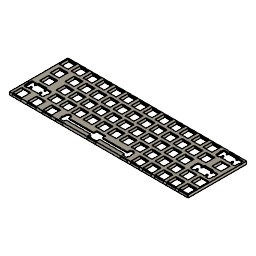
Plate (Autodesk Fusion 360 design; units mm, degrees)
Autodesk Fusion 360 part; units mm, degrees
(part 1 of 2)
sketch "b27d7a26cd9df215f168af8e672502c9323f781d_switch" plane through (0, 0, 0) normal (0, 0, 1) x (1, 0, 0)
  line L0 (271.224, 49.9939) -> (271.224, 54.6929)
  line L1 (255.699, 49.9939) -> (255.699, 53.2225)
  line L2 (248.95, 53.2225) -> (248.95, 49.9939)
  line L3 (255.699, 40.9236) -> (255.699, 45.394)
  line L4 (248.95, 47.1921) -> (248.95, 40.9236)
  line L5 (283.13, 21.6435) -> (269.131, 21.6435)
  line L6 (257.223, 40.6922) -> (271.224, 40.6922)
  line L7 (248.126, 47.1921) -> (248.95, 47.1921)
  line L8 (23.5755, 40.6922) -> (9.576, 40.6922)
  line L9 (35.7699, 40.6922) -> (35.7699, 54.6929)
  line L10 (272.749, 49.9939) -> (271.224, 49.9939)
  line L11 (68.8178, 40.6922) -> (54.8171, 40.6922)
  line L12 (206.93, 21.6435) -> (192.931, 21.6435)
  line L13 (279.499, 49.9939) -> (279.499, 53.2225)
  line L14 (280.325, 47.1921) -> (280.325, 49.9939)
  line L15 (277.774, 40.9236) -> (279.499, 40.9236)
  line L16 (277.774, 39.7221) -> (277.774, 40.9236)
  line L17 (9.576, 54.6929) -> (23.5755, 54.6929)
  line L18 (250.675, 39.7221) -> (253.974, 39.7221)
  line L19 (106.918, 54.6929) -> (106.918, 40.6922)
  line L20 (271.224, 45.394) -> (272.749, 45.394)
  line L21 (87.8678, 40.6922) -> (73.8685, 40.6922)
  line L22 (274.475, 40.9236) -> (274.475, 39.7221)
  line L23 (106.918, 40.6922) -> (92.9185, 40.6922)
  line L24 (271.224, 54.6929) -> (257.223, 54.6929)
  line L25 (253.974, 40.9236) -> (255.699, 40.9236)
  line L26 (253.974, 39.7221) -> (253.974, 40.9236)
  line L27 (274.475, 39.7221) -> (277.774, 39.7221)
  line L28 (257.223, 49.9939) -> (255.699, 49.9939)
  line L29 (272.749, 40.9236) -> (274.475, 40.9236)
  line L30 (248.95, 40.9236) -> (250.675, 40.9236)
  line L31 (68.8178, 54.6929) -> (68.8178, 40.6922)
  line L32 (250.081, 21.6435) -> (250.081, 35.6429)
  line L33 (279.499, 53.2225) -> (272.749, 53.2225)
  line L34 (279.499, 40.9236) -> (279.499, 47.1921)
  line L35 (87.8678, 54.6929) -> (87.8678, 40.6922)
  line L36 (271.224, 40.6922) -> (271.224, 45.394)
  line L37 (73.8685, 40.6922) -> (73.8685, 54.6929)
  line L38 (23.5755, 54.6929) -> (23.5755, 40.6922)
  line L39 (272.749, 45.394) -> (272.749, 40.9236)
  line L40 (264.08, 35.6429) -> (264.08, 21.6435)
  line L41 (280.325, 49.9939) -> (279.499, 49.9939)
  line L42 (225.982, 21.6435) -> (211.981, 21.6435)
  line L43 (54.8171, 54.6929) -> (68.8178, 54.6929)
  line L44 (92.9185, 54.6929) -> (106.918, 54.6929)
  line L45 (73.8685, 54.6929) -> (87.8678, 54.6929)
  line L46 (257.223, 54.6929) -> (257.223, 49.9939)
  line L47 (272.749, 53.2225) -> (272.749, 49.9939)
  line L48 (255.699, 53.2225) -> (248.95, 53.2225)
  line L49 (264.08, 21.6435) -> (250.081, 21.6435)
  line L50 (279.499, 47.1921) -> (280.325, 47.1921)
  line L51 (283.13, 35.6429) -> (283.13, 21.6435)
  line L52 (255.699, 45.394) -> (257.223, 45.394)
  line L53 (49.7692, 40.6922) -> (35.7699, 40.6922)
  line L54 (9.576, 40.6922) -> (9.576, 54.6929)
  line L55 (35.7699, 54.6929) -> (49.7692, 54.6929)
  line L56 (49.7692, 54.6929) -> (49.7692, 40.6922)
  line L57 (248.126, 49.9939) -> (248.126, 47.1921)
  line L58 (269.131, 35.6429) -> (283.13, 35.6429)
  line L59 (54.8171, 40.6922) -> (54.8171, 54.6929)
  line L60 (257.223, 45.394) -> (257.223, 40.6922)
  line L61 (250.675, 40.9236) -> (250.675, 39.7221)
  line L62 (269.131, 21.6435) -> (269.131, 35.6429)
  line L63 (248.95, 49.9939) -> (248.126, 49.9939)
  line L64 (216.455, 73.7429) -> (216.455, 59.7436)
  line L65 (258.862, 65.0709) -> (259.559, 64.7153)
  line L66 (278.368, 59.7436) -> (264.368, 59.7436)
  line L67 (23.4583, 65.6237) -> (24.0123, 65.0709)
  line L68 (126.256, 59.7436) -> (126.256, 73.7429)
  line L69 (258.309, 65.6237) -> (258.862, 65.0709)
  line L70 (216.455, 59.7436) -> (202.456, 59.7436)
  line L71 (25.4827, 64.5915) -> (26.2544, 64.7153)
  line L72 (164.356, 73.7429) -> (178.357, 73.7429)
  line L73 (178.357, 59.7436) -> (164.356, 59.7436)
  line L74 (183.406, 73.7429) -> (197.407, 73.7429)
  line L75 (183.406, 59.7436) -> (183.406, 73.7429)
  line L76 (24.7082, 64.7153) -> (25.4827, 64.5915)
  line L77 (27.9811, 67.0913) -> (27.8598, 67.8656)
  line L78 (257.954, 66.3208) -> (258.309, 65.6237)
  line L79 (264.368, 73.7429) -> (278.368, 73.7429)
  line L80 (240.556, 59.7436) -> (240.556, 73.7429)
  line L81 (240.556, 73.7429) -> (254.555, 73.7429)
  line L82 (202.456, 73.7429) -> (216.455, 73.7429)
  line L83 (26.9517, 65.0709) -> (27.5029, 65.6237)
  line L84 (221.506, 59.7436) -> (221.506, 73.7429)
  line L85 (25.4827, 69.5925) -> (24.7082, 69.4711)
  line L86 (257.831, 67.0913) -> (257.954, 66.3208)
  line L87 (258.309, 68.5631) -> (257.954, 67.8656)
  line L88 (121.205, 73.7429) -> (121.205, 59.7436)
  line L89 (221.506, 73.7429) -> (235.507, 73.7429)
  line L90 (23.1042, 67.8656) -> (22.9829, 67.0913)
  line L91 (259.559, 69.4711) -> (258.862, 69.1155)
  line L92 (235.507, 73.7429) -> (235.507, 59.7436)
  line L93 (23.4583, 68.5631) -> (23.1042, 67.8656)
  line L94 (257.954, 67.8656) -> (257.831, 67.0913)
  line L95 (235.507, 59.7436) -> (221.506, 59.7436)
  line L96 (164.356, 59.7436) -> (164.356, 73.7429)
  line L97 (159.305, 73.7429) -> (159.305, 59.7436)
  line L98 (254.555, 73.7429) -> (254.555, 59.7436)
  line L99 (24.0123, 65.0709) -> (24.7082, 64.7153)
  line L100 (26.2544, 69.4711) -> (25.4827, 69.5925)
  line L101 (26.2544, 64.7153) -> (26.9517, 65.0709)
  line L102 (27.5029, 68.5631) -> (26.9517, 69.1155)
  line L103 (258.862, 69.1155) -> (258.309, 68.5631)
  line L104 (24.0123, 69.1155) -> (23.4583, 68.5631)
  line L105 (197.407, 73.7429) -> (197.407, 59.7436)
  line L106 (24.7082, 69.4711) -> (24.0123, 69.1155)
  line L107 (178.357, 73.7429) -> (178.357, 59.7436)
  line L108 (259.559, 64.7153) -> (260.332, 64.5915)
  line L109 (23.1042, 66.3208) -> (23.4583, 65.6237)
  line L110 (251.331, 91.3239) -> (251.331, 88.0939)
  line L111 (121.205, 59.7436) -> (107.206, 59.7436)
  line L112 (254.555, 59.7436) -> (240.556, 59.7436)
  line L113 (27.8598, 67.8656) -> (27.5029, 68.5631)
  line L114 (273.605, 92.7929) -> (259.606, 92.7929)
  line L115 (197.407, 59.7436) -> (183.406, 59.7436)
  line L116 (140.257, 73.7429) -> (140.257, 59.7436)
  line L117 (261.104, 69.4711) -> (260.332, 69.5925)
  line L118 (26.9517, 69.1155) -> (26.2544, 69.4711)
  line L119 (251.331, 85.2936) -> (251.331, 79.0222)
  line L120 (276.856, 79.0222) -> (276.856, 77.8235)
  line L121 (281.88, 88.0939) -> (281.88, 91.3239)
  line L122 (35.4817, 78.7936) -> (21.4809, 78.7936)
  line L123 (258.08, 79.0222) -> (258.08, 83.494)
  line L124 (54.5317, 92.7929) -> (54.5317, 78.7936)
  line L125 (202.456, 59.7436) -> (202.456, 73.7429)
  line L126 (280.155, 79.0222) -> (281.88, 79.0222)
  line L127 (126.256, 73.7429) -> (140.257, 73.7429)
  line L128 (275.131, 88.0939) -> (273.605, 88.0939)
  line L129 (264.368, 59.7436) -> (264.368, 73.7429)
  line L130 (251.331, 79.0222) -> (253.056, 79.0222)
  line L131 (22.9829, 67.0913) -> (23.1042, 66.3208)
  line L132 (2.4309, 78.7936) -> (2.4309, 92.7929)
  line L133 (273.605, 78.7936) -> (273.605, 83.494)
  line L134 (256.355, 79.0222) -> (258.08, 79.0222)
  line L135 (107.206, 59.7436) -> (107.206, 73.7429)
  line L136 (259.606, 83.494) -> (259.606, 78.7936)
  line L137 (280.155, 77.8235) -> (280.155, 79.0222)
  line L138 (140.257, 59.7436) -> (126.256, 59.7436)
  line L139 (40.531, 92.7929) -> (54.5317, 92.7929)
  line L140 (281.88, 85.2936) -> (282.706, 85.2936)
  line L141 (278.368, 73.7429) -> (278.368, 59.7436)
  line L142 (35.4817, 92.7929) -> (35.4817, 78.7936)
  line L143 (275.131, 79.0222) -> (276.856, 79.0222)
  line L144 (256.355, 77.8235) -> (256.355, 79.0222)
  line L145 (259.606, 92.7929) -> (259.606, 88.0939)
  line L146 (21.4809, 78.7936) -> (21.4809, 92.7929)
  line L147 (145.306, 73.7429) -> (159.305, 73.7429)
  line L148 (145.306, 59.7436) -> (145.306, 73.7429)
  line L149 (27.5029, 65.6237) -> (27.8598, 66.3208)
  line L150 (27.8598, 66.3208) -> (27.9811, 67.0913)
  line L151 (282.706, 85.2936) -> (282.706, 88.0939)
  line L152 (262.354, 65.6237) -> (262.708, 66.3208)
  line L153 (54.5317, 78.7936) -> (40.531, 78.7936)
  line L154 (159.305, 59.7436) -> (145.306, 59.7436)
  line L155 (282.706, 88.0939) -> (281.88, 88.0939)
  line L156 (16.4317, 92.7929) -> (16.4317, 78.7936)
  line L157 (250.507, 88.0939) -> (250.507, 85.2936)
  line L158 (281.88, 79.0222) -> (281.88, 85.2936)
  line L159 (258.08, 91.3239) -> (251.331, 91.3239)
  line L160 (16.4317, 78.7936) -> (2.4309, 78.7936)
  line L161 (258.08, 83.494) -> (259.606, 83.494)
  line L162 (281.88, 91.3239) -> (275.131, 91.3239)
  line L163 (261.801, 65.0709) -> (262.354, 65.6237)
  line L164 (276.856, 77.8235) -> (280.155, 77.8235)
  line L165 (2.4309, 92.7929) -> (16.4317, 92.7929)
  line L166 (250.507, 85.2936) -> (251.331, 85.2936)
  line L167 (262.354, 68.5631) -> (261.801, 69.1155)
  line L168 (273.605, 83.494) -> (275.131, 83.494)
  line L169 (259.606, 88.0939) -> (258.08, 88.0939)
  line L170 (261.104, 64.7153) -> (261.801, 65.0709)
  line L171 (173.881, 92.7929) -> (187.882, 92.7929)
  line L172 (135.781, 78.7936) -> (135.781, 92.7929)
  line L173 (225.982, 78.7936) -> (211.981, 78.7936)
  line L174 (130.732, 92.7929) -> (130.732, 78.7936)
  line L175 (187.882, 78.7936) -> (173.881, 78.7936)
  line L176 (273.605, 88.0939) -> (273.605, 92.7929)
  line L177 (259.606, 78.7936) -> (273.605, 78.7936)
  line L178 (245.032, 92.7929) -> (245.032, 78.7936)
  line L179 (168.83, 92.7929) -> (168.83, 78.7936)
  line L180 (261.801, 69.1155) -> (261.104, 69.4711)
  line L181 (59.581, 78.7936) -> (59.581, 92.7929)
  line L182 (260.332, 69.5925) -> (259.559, 69.4711)
  line L183 (149.782, 78.7936) -> (135.781, 78.7936)
  line L184 (73.5803, 92.7929) -> (73.5803, 78.7936)
  line L185 (262.708, 66.3208) -> (262.832, 67.0913)
  line L186 (262.708, 67.8656) -> (262.354, 68.5631)
  line L187 (40.531, 78.7936) -> (40.531, 92.7929)
  line L188 (78.631, 78.7936) -> (78.631, 92.7929)
  line L189 (111.682, 78.7936) -> (97.681, 78.7936)
  line L190 (78.631, 92.7929) -> (92.6317, 92.7929)
  line L191 (97.681, 78.7936) -> (97.681, 92.7929)
  line L192 (21.4809, 92.7929) -> (35.4817, 92.7929)
  line L193 (59.581, 92.7929) -> (73.5803, 92.7929)
  line L194 (258.08, 88.0939) -> (258.08, 91.3239)
  line L195 (253.056, 79.0222) -> (253.056, 77.8235)
  line L196 (206.93, 78.7936) -> (192.931, 78.7936)
  line L197 (130.732, 78.7936) -> (116.731, 78.7936)
  line L198 (275.131, 91.3239) -> (275.131, 88.0939)
  line L199 (275.131, 83.494) -> (275.131, 79.0222)
  line L200 (73.5803, 78.7936) -> (59.581, 78.7936)
  line L201 (251.331, 88.0939) -> (250.507, 88.0939)
  line L202 (260.332, 64.5915) -> (261.104, 64.7153)
  line L203 (231.031, 92.7929) -> (245.032, 92.7929)
  line L204 (154.831, 92.7929) -> (168.83, 92.7929)
  line L205 (154.831, 78.7936) -> (154.831, 92.7929)
  line L206 (187.882, 92.7929) -> (187.882, 78.7936)
  line L207 (253.056, 77.8235) -> (256.355, 77.8235)
  line L208 (192.931, 92.7929) -> (206.93, 92.7929)
  line L209 (211.981, 92.7929) -> (225.982, 92.7929)
  line L210 (192.931, 78.7936) -> (192.931, 92.7929)
  line L211 (111.682, 92.7929) -> (111.682, 78.7936)
  line L212 (262.832, 67.0913) -> (262.708, 67.8656)
  line L213 (149.782, 92.7929) -> (149.782, 78.7936)
  line L214 (116.731, 92.7929) -> (130.732, 92.7929)
  line L215 (211.981, 78.7936) -> (211.981, 92.7929)
  line L216 (97.681, 92.7929) -> (111.682, 92.7929)
  line L217 (173.881, 78.7936) -> (173.881, 92.7929)
  line L218 (206.93, 92.7929) -> (206.93, 78.7936)
  line L219 (116.731, 78.7936) -> (116.731, 92.7929)
  line L220 (231.031, 78.7936) -> (231.031, 92.7929)
  line L221 (225.982, 92.7929) -> (225.982, 78.7936)
  line L222 (92.6317, 92.7929) -> (92.6317, 78.7936)
  line L223 (92.6317, 78.7936) -> (78.631, 78.7936)
  line L224 (168.83, 78.7936) -> (154.831, 78.7936)
  line L225 (135.781, 92.7929) -> (149.782, 92.7929)
  line L226 (245.032, 78.7936) -> (231.031, 78.7936)
  line L227 (50.056, 73.7429) -> (64.0567, 73.7429)
  line L228 (130.859, 46.9209) -> (130.983, 47.6913)
  line L229 (126.46, 49.1613) -> (126.103, 48.4657)
  line L230 (64.0567, 73.7429) -> (64.0567, 59.7436)
  line L231 (169.12, 54.6929) -> (183.119, 54.6929)
  line L232 (127.71, 45.314) -> (128.483, 45.1915)
  line L233 (183.119, 40.6922) -> (169.12, 40.6922)
  line L234 (125.969, 40.6922) -> (111.967, 40.6922)
  line L235 (102.157, 59.7436) -> (88.156, 59.7436)
  line L236 (145.018, 54.6929) -> (145.018, 40.6922)
  line L237 (221.219, 40.6922) -> (207.22, 40.6922)
  line L238 (21.1942, 59.7436) -> (7.1947, 59.7436)
  line L239 (128.483, 45.1915) -> (129.255, 45.314)
  line L240 (102.157, 73.7429) -> (102.157, 59.7436)
  line L241 (130.859, 48.4657) -> (130.504, 49.1613)
  line L242 (127.012, 45.671) -> (127.71, 45.314)
  line L243 (202.168, 40.6922) -> (188.168, 40.6922)
  line L244 (127.71, 50.0712) -> (127.012, 49.7156)
  line L245 (107.206, 73.7429) -> (121.205, 73.7429)
  line L246 (130.983, 47.6913) -> (130.859, 48.4657)
  line L247 (150.068, 54.6929) -> (164.068, 54.6929)
  line L248 (164.068, 40.6922) -> (150.068, 40.6922)
  line L249 (240.269, 54.6929) -> (240.269, 40.6922)
  line L250 (69.106, 59.7436) -> (69.106, 73.7429)
  line L251 (83.1067, 73.7429) -> (83.1067, 59.7436)
  line L252 (111.967, 54.6929) -> (125.969, 54.6929)
  line L253 (88.156, 59.7436) -> (88.156, 73.7429)
  line L254 (83.1067, 59.7436) -> (69.106, 59.7436)
  line L255 (88.156, 73.7429) -> (102.157, 73.7429)
  line L256 (226.27, 40.6922) -> (226.27, 54.6929)
  line L257 (131.018, 54.6929) -> (145.018, 54.6929)
  line L258 (92.9185, 40.6922) -> (92.9185, 54.6929)
  line L259 (126.103, 48.4657) -> (125.983, 47.6913)
  line L260 (31.0059, 73.7429) -> (45.0053, 73.7429)
  line L261 (50.056, 59.7436) -> (50.056, 73.7429)
  line L262 (69.106, 73.7429) -> (83.1067, 73.7429)
  line L263 (164.068, 54.6929) -> (164.068, 40.6922)
  line L264 (125.983, 47.6913) -> (126.103, 46.9209)
  line L265 (150.068, 40.6922) -> (150.068, 54.6929)
  line L266 (145.018, 40.6922) -> (131.018, 40.6922)
  line L267 (183.119, 54.6929) -> (183.119, 40.6922)
  line L268 (126.103, 46.9209) -> (126.46, 46.222)
  line L269 (130.504, 49.1613) -> (129.952, 49.7156)
  line L270 (64.0567, 59.7436) -> (50.056, 59.7436)
  line L271 (221.219, 54.6929) -> (221.219, 40.6922)
  line L272 (129.255, 50.0712) -> (128.483, 50.1908)
  line L273 (125.969, 54.6929) -> (125.969, 40.6922)
  line L274 (131.018, 40.6922) -> (131.018, 54.6929)
  line L275 (129.255, 45.314) -> (129.952, 45.671)
  line L276 (129.952, 49.7156) -> (129.255, 50.0712)
  line L277 (45.0053, 73.7429) -> (45.0053, 59.7436)
  line L278 (226.27, 54.6929) -> (240.269, 54.6929)
  line L279 (21.1942, 73.7429) -> (21.1942, 59.7436)
  line L280 (111.967, 40.6922) -> (111.967, 54.6929)
  line L281 (188.168, 40.6922) -> (188.168, 54.6929)
  line L282 (207.22, 40.6922) -> (207.22, 54.6929)
  line L283 (240.269, 40.6922) -> (226.27, 40.6922)
  line L284 (188.168, 54.6929) -> (202.168, 54.6929)
  line L285 (130.504, 46.222) -> (130.859, 46.9209)
  line L286 (127.012, 49.7156) -> (126.46, 49.1613)
  line L287 (7.1947, 59.7436) -> (7.1947, 73.7429)
  line L288 (45.0053, 59.7436) -> (31.0059, 59.7436)
  line L289 (7.1947, 73.7429) -> (21.1942, 73.7429)
  line L290 (128.483, 50.1908) -> (127.71, 50.0712)
  line L291 (5.6169, 37.0237) -> (5.971, 37.7197)
  line L292 (184.284, 16.3477) -> (182.5589, 16.3477)
  line L293 (3.5953, 40.9924) -> (0.0951, 40.9924)
  line L294 (0.0951, 95.3477) -> (285.469, 95.3477)
  line L295 (279.592, 37.7197) -> (279.947, 37.0237)
  line L296 (207.22, 54.6929) -> (221.219, 54.6929)
  line L297 (279.947, 37.0237) -> (280.5, 36.4698)
  line L298 (281.969, 40.9924) -> (281.196, 40.87)
  line L299 (279.592, 39.2659) -> (279.469, 38.4941)
  line L300 (137.909, 2.5783) -> (137.909, 7.2775)
  line L301 (281.969, 35.9929) -> (285.469, 35.9929)
  line L302 (6.095, 38.4926) -> (5.971, 39.2659)
  line L303 (285.469, 35.9929) -> (285.469, 0.2288)
  line L304 (285.469, 0.2288) -> (0.0951, 0.2288)
  line L305 (285.469, 95.3477) -> (285.469, 40.9924)
  line L306 (177.5346, 4.0473) -> (184.284, 4.0473)
  line L307 (5.6169, 39.963) -> (5.0629, 40.5158)
  line L308 (279.469, 38.4941) -> (279.592, 37.7197)
  line L309 (5.0629, 36.4698) -> (5.6169, 37.0237)
  line L310 (184.284, 4.0473) -> (184.284, 7.2775)
  line L311 (279.947, 39.963) -> (279.592, 39.2659)
  line L312 (281.196, 40.87) -> (280.5, 40.5158)
  line L313 (31.0059, 59.7436) -> (31.0059, 73.7429)
  line L314 (202.168, 54.6929) -> (202.168, 40.6922)
  line L315 (184.284, 7.2775) -> (185.1095, 7.2775)
  line L316 (280.5, 36.4698) -> (281.196, 36.1142)
  line L317 (3.5939, 35.9929) -> (4.367, 36.1142)
  line L318 (169.12, 40.6922) -> (169.12, 54.6929)
  line L319 (184.284, 10.0776) -> (184.284, 16.3477)
  line L320 (0.0951, 0.2288) -> (0.0951, 35.9929)
  line L321 (280.5, 40.5158) -> (279.947, 39.963)
  line L322 (281.196, 36.1142) -> (281.969, 35.9929)
  line L323 (0.0951, 40.9924) -> (0.0951, 95.3477)
  line L324 (4.367, 36.1142) -> (5.0629, 36.4698)
  line L325 (285.469, 40.9924) -> (281.969, 40.9924)
  line L326 (5.971, 39.2659) -> (5.6169, 39.963)
  line L327 (182.5589, 16.3477) -> (182.5589, 17.548)
  line L328 (5.971, 37.7197) -> (6.095, 38.4926)
  line L329 (129.952, 45.671) -> (130.504, 46.222)
  line L330 (126.46, 46.222) -> (127.012, 45.671)
  line L331 (137.909, 16.5778) -> (123.91, 16.5778)
  line L332 (123.91, 16.5778) -> (123.91, 11.8773)
  line L333 (84.284, 11.8773) -> (84.284, 16.3477)
  line L334 (137.909, 7.2775) -> (177.5346, 7.2775)
  line L335 (82.56, 17.548) -> (79.26, 17.548)
  line L336 (79.26, 17.548) -> (79.26, 16.3477)
  line L337 (4.367, 40.87) -> (3.5953, 40.9924)
  line L338 (77.534, 10.0776) -> (76.71, 10.0776)
  line L339 (76.71, 10.0776) -> (76.71, 7.2775)
  line L340 (84.284, 4.0473) -> (84.284, 7.2775)
  line L341 (4.8121, 16.593) -> (18.813, 16.593)
  line L342 (18.813, 16.593) -> (18.813, 2.5935)
  line L343 (4.8121, 2.5935) -> (4.8121, 16.593)
  line L344 (123.91, 2.5783) -> (137.909, 2.5783)
  line L345 (192.931, 2.5935) -> (206.93, 2.5935)
  line L346 (84.284, 16.3477) -> (82.56, 16.3477)
  line L347 (245.032, 16.593) -> (245.032, 2.5935)
  line L348 (211.981, 16.593) -> (225.982, 16.593)
  line L349 (76.71, 7.2775) -> (77.534, 7.2775)
  line L350 (77.534, 7.2775) -> (77.534, 4.0473)
  line L351 (123.91, 11.8773) -> (84.284, 11.8773)
  line L352 (177.5346, 7.2775) -> (177.5346, 4.0473)
  line L353 (77.534, 4.0473) -> (84.284, 4.0473)
  line L354 (84.284, 7.2775) -> (123.91, 7.2775)
  line L355 (18.813, 2.5935) -> (4.8121, 2.5935)
  line L356 (0.0951, 35.9929) -> (3.5939, 35.9929)
  line L357 (123.91, 7.2775) -> (123.91, 2.5783)
  line L358 (192.931, 11.0133) -> (192.804, 11.2627)
  line L359 (245.032, 2.5935) -> (231.031, 2.5935)
  line L360 (5.0629, 40.5158) -> (4.367, 40.87)
  line L361 (179.2597, 16.3477) -> (177.5346, 16.3477)
  line L362 (82.56, 16.3477) -> (82.56, 17.548)
  line L363 (137.909, 11.8773) -> (137.909, 16.5778)
  line L364 (79.26, 16.3477) -> (77.534, 16.3477)
  line L365 (177.5346, 16.3477) -> (177.5346, 11.8773)
  line L366 (77.534, 16.3477) -> (77.534, 10.0776)
  line L367 (182.5589, 17.548) -> (179.2597, 17.548)
  line L368 (179.2597, 17.548) -> (179.2597, 16.3477)
  line L369 (177.5346, 11.8773) -> (137.909, 11.8773)
  line L370 (231.031, 2.5935) -> (231.031, 16.593)
  line L371 (250.081, 2.5935) -> (250.081, 16.593)
  line L372 (269.131, 16.593) -> (283.13, 16.593)
  line L373 (269.131, 2.5935) -> (269.131, 16.593)
  line L374 (10.4317, 34.174) -> (3.6821, 34.174)
  line L375 (2.8567, 28.1437) -> (3.6821, 28.1437)
  line L376 (11.9558, 30.9425) -> (10.4317, 30.9425)
  line L377 (66.4379, 16.593) -> (66.4379, 2.5935)
  line L378 (3.6821, 28.1437) -> (3.6821, 21.8736)
  line L379 (3.6821, 21.8736) -> (5.406, 21.8736)
  line L380 (10.4317, 26.344) -> (11.9558, 26.344)
  line L381 (10.4317, 21.8736) -> (10.4317, 26.344)
  line L382 (264.08, 16.593) -> (264.08, 2.5935)
  line L383 (189.312, 7.7694) -> (190.008, 7.4152)
  line L384 (2.8567, 30.9425) -> (2.8567, 28.1437)
  line L385 (42.624, 16.593) -> (42.624, 2.5935)
  line L386 (250.081, 16.593) -> (264.08, 16.593)
  line L387 (283.13, 16.593) -> (283.13, 2.5935)
  line L388 (189.312, 11.8139) -> (188.758, 11.2627)
  line L389 (206.93, 2.5935) -> (206.93, 16.593)
  line L390 (188.758, 8.3234) -> (189.312, 7.7694)
  line L391 (5.406, 20.6733) -> (8.7065, 20.6733)
  line L392 (8.7065, 20.6733) -> (8.7065, 21.8736)
  line L393 (225.982, 2.5935) -> (211.981, 2.5935)
  line L394 (28.6246, 16.593) -> (42.624, 16.593)
  line L395 (28.6246, 2.5935) -> (28.6246, 16.593)
  line L396 (10.4317, 30.9425) -> (10.4317, 34.174)
  line L397 (11.9558, 26.344) -> (11.9558, 21.6435)
  line L398 (190.781, 12.2921) -> (190.008, 12.1708)
  line L399 (190.008, 12.1708) -> (189.312, 11.8139)
  line L400 (188.758, 11.2627) -> (188.404, 10.564)
  line L401 (192.252, 11.8139) -> (191.554, 12.1708)
  line L402 (32.5052, 20.6733) -> (32.5052, 21.8736)
  line L403 (25.9553, 30.9425) -> (25.9553, 35.6429)
  line L404 (42.624, 2.5935) -> (28.6246, 2.5935)
  line L405 (192.804, 11.2627) -> (192.252, 11.8139)
  line L406 (245.032, 21.6435) -> (231.031, 21.6435)
  line L407 (52.4372, 16.593) -> (66.4379, 16.593)
  line L408 (192.252, 7.7694) -> (192.804, 8.3234)
  line L409 (192.931, 8.5728) -> (192.931, 2.5935)
  line L410 (188.281, 9.7923) -> (188.404, 9.0193)
  line L411 (188.404, 9.0193) -> (188.758, 8.3234)
  line L412 (264.08, 2.5935) -> (250.081, 2.5935)
  line L413 (211.981, 2.5935) -> (211.981, 16.593)
  line L414 (190.008, 7.4152) -> (190.781, 7.2926)
  line L415 (8.7065, 21.8736) -> (10.4317, 21.8736)
  line L416 (191.554, 12.1708) -> (190.781, 12.2921)
  line L417 (225.982, 16.593) -> (225.982, 2.5935)
  line L418 (66.4379, 2.5935) -> (52.4372, 2.5935)
  line L419 (3.6821, 34.174) -> (3.6821, 30.9425)
  line L420 (231.031, 16.593) -> (245.032, 16.593)
  line L421 (5.406, 21.8736) -> (5.406, 20.6733)
  line L422 (283.13, 2.5935) -> (269.131, 2.5935)
  line L423 (3.6821, 30.9425) -> (2.8567, 30.9425)
  line L424 (190.781, 7.2926) -> (191.554, 7.4152)
  line L425 (192.931, 16.593) -> (192.931, 11.0133)
  line L426 (191.554, 7.4152) -> (192.252, 7.7694)
  line L427 (211.981, 21.6435) -> (211.981, 35.6429)
  line L428 (192.804, 8.3234) -> (192.931, 8.5728)
  line L429 (245.032, 35.6429) -> (245.032, 21.6435)
  line L430 (188.404, 10.564) -> (188.281, 9.7923)
  line L431 (52.4372, 2.5935) -> (52.4372, 16.593)
  line L432 (206.93, 16.593) -> (192.931, 16.593)
  line L433 (11.9558, 35.6429) -> (11.9558, 30.9425)
  line L434 (173.881, 21.6435) -> (173.881, 35.6429)
  line L435 (34.2319, 28.1437) -> (35.0559, 28.1437)
  line L436 (225.982, 35.6429) -> (225.982, 21.6435)
  line L437 (154.831, 35.6429) -> (168.83, 35.6429)
  line L438 (116.731, 21.6435) -> (116.731, 35.6429)
  line L439 (135.781, 35.6429) -> (149.782, 35.6429)
  line L440 (35.0559, 30.9425) -> (34.2319, 30.9425)
  line L441 (40.531, 21.6435) -> (40.531, 35.6429)
  line L442 (135.781, 21.6435) -> (135.781, 35.6429)
  line L443 (54.5317, 35.6429) -> (54.5317, 21.6435)
  line L444 (34.2319, 21.8736) -> (34.2319, 28.1437)
  line L445 (173.881, 35.6429) -> (187.882, 35.6429)
  line L446 (27.4808, 34.174) -> (27.4808, 30.9425)
  line L447 (73.5803, 35.6429) -> (73.5803, 21.6435)
  line L448 (231.031, 35.6429) -> (245.032, 35.6429)
  line L449 (27.4808, 26.344) -> (27.4808, 21.8736)
  line L450 (97.681, 35.6429) -> (111.682, 35.6429)
  line L451 (187.882, 21.6435) -> (173.881, 21.6435)
  line L452 (250.081, 35.6429) -> (264.08, 35.6429)
  line L453 (130.732, 21.6435) -> (116.731, 21.6435)
  line L454 (59.581, 35.6429) -> (73.5803, 35.6429)
  line L455 (73.5803, 21.6435) -> (59.581, 21.6435)
  line L456 (78.631, 35.6429) -> (92.6317, 35.6429)
  line L457 (92.6317, 21.6435) -> (78.631, 21.6435)
  line L458 (168.83, 35.6429) -> (168.83, 21.6435)
  line L459 (29.2062, 21.8736) -> (29.2062, 20.6733)
  line L460 (29.2062, 20.6733) -> (32.5052, 20.6733)
  line L461 (27.4808, 21.8736) -> (29.2062, 21.8736)
  line L462 (92.6317, 35.6429) -> (92.6317, 21.6435)
  line L463 (111.682, 35.6429) -> (111.682, 21.6435)
  line L464 (231.031, 21.6435) -> (231.031, 35.6429)
  line L465 (35.0559, 28.1437) -> (35.0559, 30.9425)
  line L466 (11.9558, 21.6435) -> (25.9553, 21.6435)
  line L467 (154.831, 21.6435) -> (154.831, 35.6429)
  line L468 (78.631, 21.6435) -> (78.631, 35.6429)
  line L469 (97.681, 21.6435) -> (97.681, 35.6429)
  line L470 (149.782, 35.6429) -> (149.782, 21.6435)
  line L471 (168.83, 21.6435) -> (154.831, 21.6435)
  line L472 (25.9553, 35.6429) -> (11.9558, 35.6429)
  line L473 (32.5052, 21.8736) -> (34.2319, 21.8736)
  line L474 (130.732, 35.6429) -> (130.732, 21.6435)
  line L475 (34.2319, 34.174) -> (27.4808, 34.174)
  line L476 (40.531, 35.6429) -> (54.5317, 35.6429)
  line L477 (192.931, 35.6429) -> (206.93, 35.6429)
  line L478 (54.5317, 21.6435) -> (40.531, 21.6435)
  line L479 (34.2319, 30.9425) -> (34.2319, 34.174)
  line L480 (25.9553, 21.6435) -> (25.9553, 26.344)
  line L481 (25.9553, 26.344) -> (27.4808, 26.344)
  line L482 (116.731, 35.6429) -> (130.732, 35.6429)
  line L483 (111.682, 21.6435) -> (97.681, 21.6435)
  line L484 (206.93, 35.6429) -> (206.93, 21.6435)
  line L485 (192.931, 21.6435) -> (192.931, 35.6429)
  line L486 (149.782, 21.6435) -> (135.781, 21.6435)
  line L487 (27.4808, 30.9425) -> (25.9553, 30.9425)
  line L488 (211.981, 35.6429) -> (225.982, 35.6429)
  line L489 (187.882, 35.6429) -> (187.882, 21.6435)
  line L490 (59.581, 21.6435) -> (59.581, 35.6429)
  line L491 (0.0951, 40.9924) -> (0.0951, 35.9929)
  line L492 (285.469, 40.9924) -> (285.469, 35.9929)
  line L493 (0.0951, 93.7929) -> (285.469, 93.7929)
  line L494 (0.0951, 77.2936) -> (285.469, 77.2936)
  line L495 (285.469, 75.2429) -> (0.0951, 75.2429)
  line L496 (0.0951, 58.2436) -> (285.469, 58.2436)
  line L497 (285.469, 56.1929) -> (0.0951, 56.1929)
  line L498 (0.0951, 39.1922) -> (285.469, 39.1922)
  line L499 (285.469, 37.1429) -> (0.0951, 37.1429)
  line L500 (0.0951, 18.093) -> (285.469, 18.093)
  line L501 (285.469, 20.1435) -> (0.0951, 20.1435)
  line L502 (0.0951, 1.5935) -> (285.469, 1.5935)
  line L503 (16.4317, 93.7929) -> (16.4317, 77.2936)
  line L504 (21.4809, 93.7929) -> (21.4809, 77.2936)
  line L505 (35.4817, 93.7929) -> (35.4817, 77.2936)
  line L506 (40.531, 93.7929) -> (40.531, 77.2936)
  line L507 (54.5317, 93.7929) -> (54.5317, 77.2936)
  line L508 (59.581, 93.7929) -> (59.581, 77.2936)
  line L509 (73.5803, 93.7929) -> (73.5803, 77.2936)
  line L510 (78.631, 93.7929) -> (78.631, 77.2936)
  line L511 (92.6317, 93.7929) -> (92.6317, 77.2936)
  line L512 (97.681, 93.7929) -> (97.681, 77.2936)
  line L513 (111.682, 93.7929) -> (111.682, 77.2936)
  line L514 (116.731, 93.7929) -> (116.731, 77.2936)
  line L515 (130.732, 93.7929) -> (130.732, 77.2936)
  line L516 (135.781, 93.7929) -> (135.781, 77.2936)
  line L517 (149.782, 93.7929) -> (149.782, 77.2936)
  line L518 (154.831, 93.7929) -> (154.831, 77.2936)
  line L519 (168.83, 93.7929) -> (168.83, 77.2936)
  line L520 (173.881, 93.7929) -> (173.881, 77.2936)
  line L521 (187.882, 93.7929) -> (187.882, 77.2936)
  line L522 (192.931, 93.7929) -> (192.931, 77.2936)
  line L523 (206.93, 93.7929) -> (206.93, 77.2936)
  line L524 (211.981, 93.7929) -> (211.981, 77.2936)
  line L525 (225.982, 93.7929) -> (225.982, 77.2936)
  line L526 (231.031, 93.7929) -> (231.031, 77.2936)
  line L527 (245.032, 93.7929) -> (245.032, 77.2936)
  line L528 (278.368, 75.2429) -> (278.368, 58.2436)
  line L529 (264.368, 75.2429) -> (264.368, 58.2436)
  line L530 (254.555, 75.2429) -> (254.555, 58.2436)
  line L531 (240.556, 75.2429) -> (240.556, 58.2436)
  line L532 (235.507, 75.2429) -> (235.507, 58.2436)
  line L533 (221.506, 75.2429) -> (221.506, 58.2436)
  line L534 (216.455, 75.2429) -> (216.455, 58.2436)
  line L535 (202.456, 75.2429) -> (202.456, 58.2436)
  line L536 (197.407, 75.2429) -> (197.407, 58.2436)
  line L537 (183.406, 75.2429) -> (183.406, 58.2436)
  line L538 (178.357, 75.2429) -> (178.357, 58.2436)
  line L539 (164.356, 75.2429) -> (164.356, 58.2436)
  line L540 (159.305, 75.2429) -> (159.305, 58.2436)
  line L541 (145.306, 75.2429) -> (145.306, 58.2436)
  line L542 (140.257, 75.2429) -> (140.257, 58.2436)
  line L543 (126.256, 75.2429) -> (126.256, 58.2436)
  line L544 (121.205, 75.2429) -> (121.205, 58.2436)
  line L545 (107.206, 75.2429) -> (107.206, 58.2436)
  line L546 (88.156, 75.2429) -> (88.156, 58.2436)
  line L547 (83.1067, 75.2429) -> (83.1067, 58.2436)
  line L548 (69.106, 75.2429) -> (69.106, 58.2436)
  line L549 (64.0567, 75.2429) -> (64.0567, 58.2436)
  line L550 (50.056, 75.2429) -> (50.056, 58.2436)
  line L551 (45.0053, 75.2429) -> (45.0053, 58.2436)
  line L552 (31.0059, 75.2429) -> (31.0059, 58.2436)
  line L553 (21.1942, 75.2429) -> (21.1942, 58.2436)
  line L554 (7.1947, 75.2429) -> (7.1947, 58.2436)
  line L555 (9.576, 56.1929) -> (9.576, 39.1922)
  line L556 (23.5755, 56.1929) -> (23.5755, 39.1922)
  line L557 (35.7699, 56.1929) -> (35.7699, 39.1922)
  line L558 (49.7692, 56.1929) -> (49.7692, 39.1922)
  line L559 (54.8171, 56.1929) -> (54.8171, 39.1922)
  line L560 (68.8178, 56.1929) -> (68.8178, 39.1922)
  line L561 (73.8685, 56.1929) -> (73.8685, 39.1922)
  line L562 (87.8678, 56.1929) -> (87.8678, 39.1922)
  line L563 (92.9185, 56.1929) -> (92.9185, 39.1922)
  line L564 (106.918, 56.1929) -> (106.918, 39.1922)
  line L565 (111.967, 56.1929) -> (111.967, 39.1922)
  line L566 (125.969, 56.1929) -> (125.969, 39.1922)
  line L567 (131.018, 56.1929) -> (131.018, 39.1922)
  line L568 (145.018, 56.1929) -> (145.018, 39.1922)
  line L569 (150.068, 56.1929) -> (150.068, 39.1922)
  line L570 (164.068, 56.1929) -> (164.068, 39.1922)
  line L571 (169.12, 56.1929) -> (169.12, 39.1922)
  line L572 (183.119, 56.1929) -> (183.119, 39.1922)
  line L573 (188.168, 56.1929) -> (188.168, 39.1922)
  line L574 (202.168, 56.1929) -> (202.168, 39.1922)
  line L575 (207.22, 56.1929) -> (207.22, 39.1922)
  line L576 (221.219, 56.1929) -> (221.219, 39.1922)
  line L577 (226.27, 56.1929) -> (226.27, 39.1922)
  line L578 (240.269, 56.1929) -> (240.269, 39.1922)
  line L579 (283.13, 37.1429) -> (283.13, 20.1435)
  line L580 (269.131, 37.1429) -> (269.131, 20.1435)
  line L581 (264.08, 37.1429) -> (264.08, 20.1435)
  line L582 (250.081, 37.1429) -> (250.081, 20.1435)
  line L583 (245.032, 37.1429) -> (245.032, 20.1435)
  line L584 (231.031, 37.1429) -> (231.031, 20.1435)
  line L585 (225.982, 37.1429) -> (225.982, 20.1435)
  line L586 (211.981, 37.1429) -> (211.981, 20.1435)
  line L587 (206.93, 37.1429) -> (206.93, 20.1435)
  line L588 (192.931, 37.1429) -> (192.931, 20.1435)
  line L589 (187.882, 37.1429) -> (187.882, 20.1435)
  line L590 (173.881, 37.1429) -> (173.881, 20.1435)
  line L591 (168.83, 37.1429) -> (168.83, 20.1435)
  line L592 (154.831, 37.1429) -> (154.831, 20.1435)
  line L593 (149.782, 37.1429) -> (149.782, 20.1435)
  line L594 (135.781, 37.1429) -> (135.781, 20.1435)
  line L595 (130.732, 37.1429) -> (130.732, 20.1435)
  line L596 (116.731, 37.1429) -> (116.731, 20.1435)
  line L597 (111.682, 37.1429) -> (111.682, 20.1435)
  line L598 (97.681, 37.1429) -> (97.681, 20.1435)
  line L599 (92.6317, 37.1429) -> (92.6317, 20.1435)
  line L600 (78.631, 37.1429) -> (78.631, 20.1435)
  line L601 (73.5803, 37.1429) -> (73.5803, 20.1435)
  line L602 (59.581, 37.1429) -> (59.581, 20.1435)
  line L603 (54.5317, 37.1429) -> (54.5317, 20.1435)
  line L604 (40.531, 37.1429) -> (40.531, 20.1435)
  line L605 (4.8121, 18.093) -> (4.8121, 1.5935)
  line L606 (18.813, 18.093) -> (18.813, 1.5935)
  line L607 (28.6246, 18.093) -> (28.6246, 1.5935)
  line L608 (42.624, 18.093) -> (42.624, 1.5935)
  line L609 (52.4372, 18.093) -> (52.4372, 1.5935)
  line L610 (66.4379, 18.093) -> (66.4379, 1.5935)
  line L611 (192.931, 18.093) -> (192.931, 1.5935)
  line L612 (206.93, 18.093) -> (206.93, 1.5935)
  line L613 (211.981, 18.093) -> (211.981, 1.5935)
  line L614 (225.982, 18.093) -> (225.982, 1.5935)
  line L615 (231.031, 18.093) -> (231.031, 1.0935)
  line L616 (245.032, 18.093) -> (245.032, 1.0935)
  line L617 (250.081, 18.093) -> (250.081, 1.5935)
  line L618 (264.08, 18.093) -> (264.08, 1.5935)
  line L619 (269.131, 18.093) -> (269.131, 1.0935)
  line L620 (283.13, 18.093) -> (283.13, 1.5935)
  line L621 (123.91, 2.5783) -> (137.909, 16.5778) construction
  line L622 (137.909, 2.5783) -> (123.91, 16.5778) construction
  circle A0 centre (130.8755, 9.5932) radius 2.8886 construction
  line L623 (185.1095, 7.2775) -> (185.1095, 11.5) construction
  line L624 (184.284, 10.0776) -> (185.1095, 10.0776)
  line L625 (185.1095, 7.2775) -> (185.1095, 10.0776)
  line L626 (85.3237, 1.5935) -> (85.3237, 7.2775)
  line L627 (123.91, 2.5783) -> (123.91, 1.5935)
  line L628 (137.909, 2.5783) -> (137.909, 1.5935)
  line L629 (176.5478, 7.2775) -> (176.5478, 1.5935)
  line L630 (187.882, 20.1435) -> (187.882, 1.5935)
  line L631 (73.5803, 20.1435) -> (73.5803, 1.0935)
  line L632 (2.4309, 93.7929) -> (2.4309, 77.2936)
  line L633 (73.5803, 21.6435) -> (173.881, 21.6435)
  line L634 (245.032, 37.1429) -> (245.032, 39.1922)
  line L635 (283.13, 37.1429) -> (283.13, 56.1929)
  line L636 (245.032, 39.1922) -> (245.032, 56.1929)
  line L637 (283.13, 77.2936) -> (283.13, 93.7929)
  line L638 (249, 93.7929) -> (249, 77.2936)
  line L639 (35.9538, 37.1429) -> (35.9538, 18.093)
  line L640 (2.0385, 37.1429) -> (2.0385, 20.1435)
  line L641 (2.0385, 20.1435) -> (2.0385, 18.093)
  line L642 (249, 77.2936) -> (249, 75.2429)
  line L643 (283.13, 77.2936) -> (283.13, 75.2429)
  line L644 (102.157, 75.2429) -> (102.157, 58.2436)
  dimension "d1" = 1
  dimension "d2" = 1.5
  dimension "d3" = 1.5
  dimension "d4" = 1.5
  dimension "d5" = 1.5
  dimension "d6" = 1.5
  dimension "d7" = 1.5
  dimension "d8" = 1.5
  dimension "d9" = 1.5
  dimension "d10" = 1
  dimension "d39" = -25
  dimension "d40" = 0
  dimension "d41" = -20
  dimension "d42" = 0
  constraint perpendicular L356 L491
  constraint perpendicular L301 L492
  constraint coincident L323 L493.start
  constraint coincident L305 L493.end
  constraint perpendicular L305 L493
  constraint coincident L323 L494.start
  constraint coincident L305 L494.end
  constraint perpendicular L305 L494
  constraint coincident L305 L495.start
  constraint coincident L323 L495.end
  constraint perpendicular L323 L495
  constraint coincident L323 L496.start
  constraint coincident L305 L496.end
  constraint perpendicular L305 L496
  constraint coincident L305 L497.start
  constraint coincident L323 L497.end
  constraint perpendicular L323 L497
  constraint coincident L491 L498.start
  constraint coincident L492 L498.end
  constraint perpendicular L492 L498
  constraint coincident L492 L499.start
  constraint coincident L491 L499.end
  constraint perpendicular L491 L499
  constraint coincident L320 L500.start
  constraint coincident L303 L500.end
  constraint perpendicular L303 L500
  constraint coincident L303 L501.start
  constraint coincident L320 L501.end
  constraint perpendicular L320 L501
  constraint coincident L320 L502.start
  constraint coincident L303 L502.end
  constraint perpendicular L303 L502
  constraint coincident L493 L503.start
  constraint coincident L494 L503.end
  constraint perpendicular L494 L503
  constraint coincident L493 L504.start
  constraint coincident L494 L504.end
  constraint perpendicular L494 L504
  constraint coincident L493 L505.start
  constraint coincident L494 L505.end
  constraint perpendicular L494 L505
  constraint coincident L493 L506.start
  constraint coincident L494 L506.end
  constraint perpendicular L494 L506
  constraint coincident L493 L507.start
  constraint coincident L494 L507.end
  constraint perpendicular L494 L507
  constraint coincident L493 L508.start
  constraint coincident L494 L508.end
  constraint perpendicular L494 L508
  constraint coincident L493 L509.start
  constraint coincident L494 L509.end
  constraint perpendicular L494 L509
  constraint coincident L493 L510.start
  constraint coincident L494 L510.end
  constraint perpendicular L494 L510
  constraint coincident L493 L511.start
  constraint coincident L494 L511.end
  constraint perpendicular L494 L511
  constraint coincident L493 L512.start
  constraint coincident L494 L512.end
  constraint perpendicular L494 L512
  constraint coincident L493 L513.start
  constraint coincident L494 L513.end
  constraint perpendicular L494 L513
  constraint coincident L493 L514.start
  constraint coincident L494 L514.end
  constraint perpendicular L494 L514
  constraint coincident L493 L515.start
  constraint coincident L494 L515.end
  constraint perpendicular L494 L515
  constraint coincident L493 L516.start
  constraint coincident L494 L516.end
  constraint perpendicular L494 L516
  constraint coincident L493 L517.start
  constraint coincident L494 L517.end
  constraint perpendicular L494 L517
  constraint coincident L493 L518.start
  constraint coincident L494 L518.end
  constraint perpendicular L494 L518
  constraint coincident L493 L519.start
  constraint coincident L494 L519.end
  constraint perpendicular L494 L519
  constraint coincident L493 L520.start
  constraint coincident L494 L520.end
  constraint perpendicular L494 L520
  constraint coincident L493 L521.start
  constraint coincident L494 L521.end
  constraint perpendicular L494 L521
  constraint coincident L493 L522.start
  constraint coincident L494 L522.end
  constraint perpendicular L494 L522
  constraint coincident L493 L523.start
  constraint coincident L494 L523.end
  constraint perpendicular L494 L523
  constraint coincident L493 L524.start
  constraint coincident L494 L524.end
  constraint perpendicular L494 L524
  constraint coincident L493 L525.start
  constraint coincident L494 L525.end
  constraint perpendicular L494 L525
  constraint coincident L493 L526.start
  constraint coincident L494 L526.end
  constraint perpendicular L494 L526
  constraint coincident L493 L527.start
  constraint coincident L494 L527.end
  constraint perpendicular L494 L527
  constraint coincident L495 L528.start
  constraint coincident L496 L528.end
  constraint perpendicular L496 L528
  constraint coincident L495 L529.start
  constraint coincident L496 L529.end
  constraint perpendicular L496 L529
  constraint coincident L495 L530.start
  constraint coincident L496 L530.end
  constraint perpendicular L496 L530
  constraint coincident L495 L531.start
  constraint coincident L496 L531.end
  constraint perpendicular L496 L531
  constraint coincident L495 L532.start
  constraint coincident L496 L532.end
  constraint perpendicular L496 L532
  constraint coincident L495 L533.start
  constraint coincident L496 L533.end
  constraint perpendicular L496 L533
  constraint coincident L495 L534.start
  constraint coincident L496 L534.end
  constraint perpendicular L496 L534
  constraint coincident L495 L535.start
  constraint coincident L496 L535.end
  constraint perpendicular L496 L535
  constraint coincident L495 L536.start
  constraint coincident L496 L536.end
  constraint perpendicular L496 L536
  constraint coincident L495 L537.start
  constraint coincident L496 L537.end
  constraint perpendicular L496 L537
  constraint coincident L495 L538.start
  constraint coincident L496 L538.end
  constraint perpendicular L496 L538
  constraint coincident L495 L539.start
  constraint coincident L496 L539.end
  constraint perpendicular L496 L539
  constraint coincident L495 L540.start
  constraint perpendicular L496 L540
  constraint coincident L495 L541.start
  constraint coincident L496 L541.end
  constraint perpendicular L496 L541
  constraint coincident L495 L542.start
  constraint perpendicular L496 L542
  constraint coincident L495 L543.start
  constraint coincident L496 L543.end
  constraint perpendicular L496 L543
  constraint coincident L495 L544.start
  constraint coincident L496 L544.end
  constraint perpendicular L496 L544
  constraint coincident L495 L545.start
  constraint coincident L496 L545.end
  constraint perpendicular L496 L545
  constraint coincident L495 L546.start
  constraint coincident L496 L546.end
  constraint perpendicular L496 L546
  constraint coincident L495 L547.start
  constraint coincident L496 L547.end
  constraint perpendicular L496 L547
  constraint coincident L495 L548.start
  constraint coincident L496 L548.end
  constraint perpendicular L496 L548
  constraint coincident L495 L549.start
  constraint coincident L496 L549.end
  constraint perpendicular L496 L549
  constraint coincident L495 L550.start
  constraint coincident L496 L550.end
  constraint perpendicular L496 L550
  constraint coincident L495 L551.start
  constraint coincident L496 L551.end
  constraint perpendicular L496 L551
  constraint coincident L495 L552.start
  constraint coincident L496 L552.end
  constraint perpendicular L496 L552
  constraint coincident L495 L553.start
  constraint coincident L496 L553.end
  constraint perpendicular L496 L553
  constraint coincident L495 L554.start
  constraint coincident L496 L554.end
  constraint perpendicular L496 L554
  constraint coincident L497 L555.start
  constraint coincident L498 L555.end
  constraint perpendicular L498 L555
  constraint coincident L497 L556.start
  constraint coincident L498 L556.end
  constraint perpendicular L498 L556
  constraint coincident L497 L557.start
  constraint coincident L498 L557.end
  constraint perpendicular L498 L557
  constraint coincident L497 L558.start
  constraint coincident L498 L558.end
  constraint perpendicular L498 L558
  constraint coincident L497 L559.start
  constraint coincident L498 L559.end
  constraint perpendicular L498 L559
  constraint coincident L497 L560.start
  constraint coincident L498 L560.end
  constraint perpendicular L498 L560
  constraint coincident L497 L561.start
  constraint coincident L498 L561.end
  constraint perpendicular L498 L561
  constraint coincident L497 L562.start
  constraint coincident L498 L562.end
  constraint perpendicular L498 L562
  constraint coincident L497 L563.start
  constraint coincident L498 L563.end
  constraint perpendicular L498 L563
  constraint coincident L497 L564.start
  constraint coincident L498 L564.end
  constraint perpendicular L498 L564
  constraint coincident L497 L565.start
  constraint coincident L498 L565.end
  constraint perpendicular L498 L565
  constraint coincident L497 L566.start
  constraint coincident L498 L566.end
  constraint perpendicular L498 L566
  constraint coincident L497 L567.start
  constraint coincident L498 L567.end
  constraint perpendicular L498 L567
  constraint coincident L497 L568.start
  constraint coincident L498 L568.end
  constraint perpendicular L498 L568
  constraint coincident L497 L569.start
  constraint coincident L498 L569.end
  constraint perpendicular L498 L569
  constraint coincident L497 L570.start
  constraint coincident L498 L570.end
  constraint perpendicular L498 L570
  constraint coincident L497 L571.start
  constraint coincident L498 L571.end
  constraint perpendicular L498 L571
  constraint coincident L497 L572.start
  constraint coincident L498 L572.end
  constraint perpendicular L498 L572
  constraint coincident L497 L573.start
  constraint perpendicular L498 L573
  constraint coincident L497 L574.start
  constraint coincident L498 L574.end
  constraint perpendicular L498 L574
  constraint coincident L497 L575.start
  constraint coincident L498 L575.end
  constraint perpendicular L498 L575
  constraint coincident L497 L576.start
  constraint coincident L498 L576.end
  constraint perpendicular L498 L576
  constraint coincident L497 L577.start
  constraint coincident L498 L577.end
  constraint perpendicular L498 L577
  constraint coincident L497 L578.start
  constraint coincident L498 L578.end
  constraint perpendicular L498 L578
  constraint coincident L499 L579.start
  constraint coincident L501 L579.end
  constraint perpendicular L501 L579
  constraint coincident L499 L580.start
  constraint coincident L501 L580.end
  constraint perpendicular L501 L580
  constraint coincident L499 L581.start
  constraint coincident L501 L581.end
  constraint perpendicular L501 L581
  constraint coincident L499 L582.start
  constraint coincident L501 L582.end
  constraint perpendicular L501 L582
  constraint coincident L499 L583.start
  constraint coincident L501 L583.end
  constraint perpendicular L501 L583
  constraint coincident L499 L584.start
  constraint coincident L501 L584.end
  constraint perpendicular L501 L584
  constraint coincident L499 L585.start
  constraint coincident L501 L585.end
  constraint perpendicular L501 L585
  constraint coincident L499 L586.start
  constraint coincident L501 L586.end
  constraint perpendicular L501 L586
  constraint coincident L499 L587.start
  constraint coincident L501 L587.end
  constraint perpendicular L501 L587
  constraint coincident L499 L588.start
  constraint coincident L501 L588.end
  constraint perpendicular L501 L588
  constraint coincident L499 L589.start
  constraint coincident L501 L589.end
  constraint perpendicular L501 L589
  constraint coincident L499 L590.start
  constraint coincident L501 L590.end
  constraint perpendicular L501 L590
  constraint coincident L499 L591.start
  constraint coincident L501 L591.end
  constraint perpendicular L501 L591
  constraint coincident L499 L592.start
  constraint coincident L501 L592.end
  constraint perpendicular L501 L592
  constraint coincident L499 L593.start
  constraint coincident L501 L593.end
  constraint perpendicular L501 L593
  constraint coincident L499 L594.start
  constraint coincident L501 L594.end
  constraint perpendicular L501 L594
  constraint coincident L499 L595.start
  constraint coincident L501 L595.end
  constraint perpendicular L501 L595
  constraint coincident L499 L596.start
  constraint coincident L501 L596.end
  constraint perpendicular L501 L596
  constraint coincident L499 L597.start
  constraint coincident L501 L597.end
  constraint perpendicular L501 L597
  constraint coincident L499 L598.start
  constraint coincident L501 L598.end
  constraint perpendicular L501 L598
  constraint coincident L499 L599.start
  constraint coincident L501 L599.end
  constraint perpendicular L501 L599
  constraint coincident L499 L600.start
  constraint coincident L501 L600.end
  constraint perpendicular L501 L600
  constraint coincident L499 L601.start
  constraint coincident L501 L601.end
  constraint perpendicular L501 L601
  constraint coincident L499 L602.start
  constraint coincident L501 L602.end
  constraint perpendicular L501 L602
  constraint coincident L499 L603.start
  constraint coincident L501 L603.end
  constraint perpendicular L501 L603
  constraint coincident L499 L604.start
  constraint coincident L501 L604.end
  constraint perpendicular L501 L604
  constraint coincident L500 L605.start
  constraint coincident L502 L605.end
  constraint perpendicular L502 L605
  constraint coincident L500 L606.start
  constraint coincident L502 L606.end
  constraint perpendicular L502 L606
  constraint coincident L500 L607.start
  constraint coincident L502 L607.end
  constraint perpendicular L502 L607
  constraint coincident L500 L608.start
  constraint coincident L502 L608.end
  constraint perpendicular L502 L608
  constraint coincident L500 L609.start
  constraint coincident L502 L609.end
  constraint perpendicular L502 L609
  constraint coincident L500 L610.start
  constraint coincident L502 L610.end
  constraint perpendicular L502 L610
  constraint coincident L500 L611.start
  constraint coincident L502 L611.end
  constraint perpendicular L502 L611
  constraint coincident L500 L612.start
  constraint coincident L502 L612.end
  constraint perpendicular L502 L612
  constraint coincident L500 L613.start
  constraint coincident L502 L613.end
  constraint perpendicular L502 L613
  constraint coincident L500 L614.start
  constraint coincident L502 L614.end
  constraint perpendicular L502 L614
  constraint coincident L500 L615.start
  constraint perpendicular L502 L615
  constraint coincident L500 L616.start
  constraint perpendicular L502 L616
  constraint coincident L500 L617.start
  constraint coincident L502 L617.end
  constraint perpendicular L502 L617
  constraint coincident L500 L618.start
  constraint coincident L502 L618.end
  constraint perpendicular L502 L618
  constraint coincident L500 L619.start
  constraint perpendicular L502 L619
  constraint coincident L500 L620.start
  constraint coincident L502 L620.end
  constraint perpendicular L502 L620
  constraint perpendicular L315 L623
  constraint coincident L623 L624.end
  constraint perpendicular L623 L624
  constraint coincident L502 L626.start
  constraint coincident L354 L626.end
  constraint perpendicular L354 L626
  constraint coincident L502 L627.end
  constraint perpendicular L502 L627
  constraint coincident L502 L628.end
  constraint perpendicular L502 L628
  constraint coincident L334 L629.start
  constraint coincident L502 L629.end
  constraint perpendicular L502 L629
  constraint coincident L502 L630.end
  constraint perpendicular L502 L630
  constraint perpendicular L502 L631
  constraint coincident L493 L632.start
  constraint coincident L494 L632.end
  constraint perpendicular L494 L632
  constraint coincident L498 L634.end
  constraint perpendicular L498 L634
  constraint coincident L497 L635.end
  constraint perpendicular L497 L635
  constraint coincident L497 L636.end
  constraint perpendicular L497 L636
  constraint coincident L494 L637.start
  constraint coincident L493 L637.end
  constraint perpendicular L493 L637
  constraint coincident L493 L638.start
  constraint coincident L494 L638.end
  constraint perpendicular L494 L638
  constraint coincident L499 L639.start